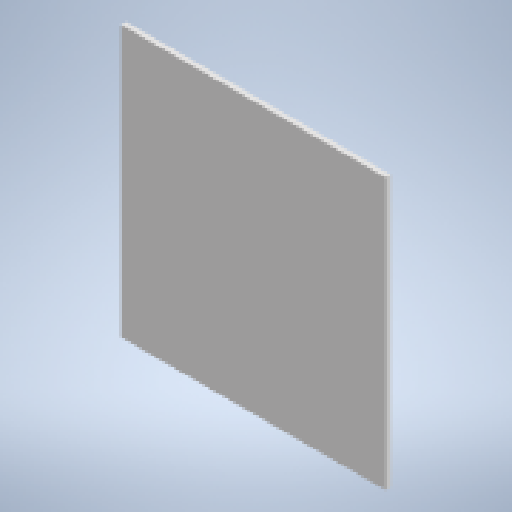
# Autodesk Inventor part: Part7
Saved by Autodesk Inventor 2023 (Build 270158000, 158)
## iProperties
Created: 2024-03-19
Part Number: Part7
Material: Generic
Document SubType Name: Modeling
Designer: noname
Density: 1 g/cm^3
Appearance: Default
Author: noname
Autodesk Inventor part; units mm, degrees
ref_plane "YZ Plane" through (0, 0, 0) normal (1, 0, 0) x (0, 1, 0)
ref_plane "XZ Plane" through (0, 0, 0) normal (0, 1, 0) x (-1, 0, 0)
ref_plane "XY Plane" through (0, 0, 0) normal (0, 0, 1) x (1, 0, 0)
sketch "Sketch1" plane through (0, 0, 0) normal (0, 0, 1) x (1, 0, 0)
  line L0 (-41.5, 42.5) -> (-41.5, -45.5) projected
  line L1 (-41.5, -45.5) -> (41.5, -45.5) projected
  line L2 (41.5, -45.5) -> (41.5, 42.5) projected
  line L3 (41.5, 42.5) -> (-41.5, 42.5) projected
  line L4 (-30.5, -35) -> (-33.5, -35) projected
  line L5 (-33.5, -35) -> (-33.5, 32) projected
  line L6 (-33.5, 32) -> (-30.5, 32) projected
  line L7 (-30.5, 32) -> (-30.5, -35) projected
  line L8 (-14.5, -35) -> (-17.5, -35) projected
  line L9 (-17.5, -35) -> (-17.5, 32) projected
  line L10 (-17.5, 32) -> (-14.5, 32) projected
  line L11 (-14.5, 32) -> (-14.5, -35) projected
  line L12 (1.5, -35) -> (-1.5, -35) projected
  line L13 (-1.5, -35) -> (-1.5, 32) projected
  line L14 (-1.5, 32) -> (1.5, 32) projected
  line L15 (1.5, 32) -> (1.5, -35) projected
  line L16 (17.5, -35) -> (14.5, -35) projected
  line L17 (14.5, -35) -> (14.5, 32) projected
  line L18 (14.5, 32) -> (17.5, 32) projected
  line L19 (17.5, 32) -> (17.5, -35) projected
  line L20 (33.5, -35) -> (30.5, -35) projected
  line L21 (30.5, -35) -> (30.5, 32) projected
  line L22 (30.5, 32) -> (33.5, 32) projected
  line L23 (33.5, 32) -> (33.5, -35) projected
  line L24 (-41.5, 42.5) -> (41.5, 42.5)
  line L25 (41.5, 42.5) -> (41.5, -57.5)
  line L26 (41.5, -57.5) -> (-41.5, -57.5)
  line L27 (-41.5, -57.5) -> (-41.5, 42.5)
  point P0 (0, 0)
  point P1 (41.5, -45.5)
  point P2 (-41.5, -45.5)
  dimension "d0" = 100
  constraints: 8 end point, 2 parallel, 1 horizontal, 1 perpendicular
  measures "d0" distance between parallel lines of L26 L3
extrude "Extrusion1" add sketch "Sketch1" along normal blind 1.6 contours L3 L2 L1 L0 | L1 L25 L26 L27 | L4 L5 L6 L7 | L8 L9 L10 L11 | L12 L13 L14 L15 | L16 L17 L18 L19 | L20 L21 L22 L23
body "Solid1"
